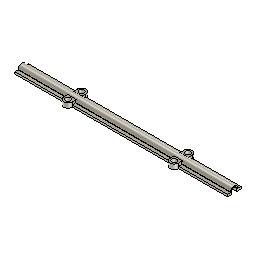
CAN_Cable_Cover v3 (Autodesk Fusion 360 design; units mm, degrees)
Autodesk Fusion 360 part; units mm, degrees
note: some values were not read from the file. Set by a fixed rule: which sketch regions a step uses.
sketch "Sketch1" plane through (0, 0, 0) normal (1, 0, 0) x (0, 1, 0) in component "CAN_Cable_Cover"
  circle A0 centre (0, 2.4) radius 2.4
  line L0 (-2.4, 2.4) -> (-2.4, 0)
  line L1 (0, 2.5) -> (0, 20)
  line L2 (2.4, 2.4) -> (2.4, 0)
  circle A1 centre (0, 2.4) radius 3.4
  line L3 (-3.4, 2.4) -> (-3.4, 0)
  line L4 (-3.4, 0) -> (-2.4, 0)
  line L5 (3.4, 2.4) -> (3.4, 0)
  line L6 (3.4, 0) -> (2.4, 0)
  line L7 (-3.4, 0) -> (-6.4, 0)
  line L8 (-6.4, 0) -> (-6.4, 2)
  line L9 (-6.4, 2) -> (-3.4, 2)
  line L10 (-3.4, 2) -> (-3.4, 0)
  line L11 (6.4, 2) -> (3.4, 2)
  line L12 (6.4, 0) -> (6.4, 2)
  line L13 (3.4, 0) -> (6.4, 0)
  line L14 (3.4, 2) -> (3.4, 0)
  dimension "d1" = 4.8
  dimension "d2" = 1
  dimension "d5" = 3
  dimension "d6" = 2
  constraint vertical origin A0.centre
  constraint coincident origin A0
  constraint coincident A0 L0.start
  constraint tangent A0 L0
  constraint vertical L0
  constraint symmetric L0.start L1 L2.start
  constraint symmetric L0.end L1 L2.end
  constraint coincident A1 L3.start
  constraint tangent A1 L3
  constraint parallel L0 L3
  constraint perpendicular L0 L4
  constraint symmetric L1 L3.start L5.start
  constraint symmetric L1 L3.end L5.end
  constraint horizontal L7
  constraint vertical L8
  constraint horizontal L9
  constraint vertical L10
  constraint symmetric L1 L7.end L12.start
  constraint symmetric L1 L8.end L11.start
  constraint symmetric L1 L9.end L11.end
  measures "d1" diameter of A0
  measures "d5" distance of L3.end L7.end
  measures "d6" distance of L3.end L9.end
extrude "Extrude1" add sketch "Sketch1" along normal mid plane 200 contours A0 L0 L1 A1 L4 | A0 L1 L2 A1 L6 | A1 L3 L4 L10 | A1 L5 L6 L14 | L3 L7 L8 L9 L10 | L5 L11 L12 L13 L14 in component "CAN_Cable_Cover"
sketch "Sketch2" plane through (0, 0, 0) normal (0, 0, -1) x (1, 0, 0) in component "CAN_Cable_Cover"
  line L0 (-100, 2.4) -> (100, 2.4)
  line L1 (100, 2.4) -> (100, 6.4)
  line L2 (100, 6.4) -> (-100, 6.4)
  line L3 (-100, 6.4) -> (-100, 2.4)
  circle A0 centre (-50, 6.4) radius 4
  line L4 (0, -1.75) -> (0, -22.5)
  circle A1 centre (-50, 6.4) radius 2.35
  line L5 (-46, 6.4) -> (-46, 2.4)
  line L6 (-46, 2.4) -> (-50, 2.4)
  line L7 (-54, 6.4) -> (-54, 2.4)
  line L8 (-54, 2.4) -> (-50, 2.4)
  line L9 (1.75, 0) -> (22.5, 0)
  circle A2 centre (-50, -6.4) radius 4
  circle A3 centre (-50, -6.4) radius 2.35
  line L10 (-54, -6.4) -> (-54, -2.4)
  line L11 (-54, -2.4) -> (-50, -2.4)
  line L12 (-46, -2.4) -> (-50, -2.4)
  line L13 (-46, -6.4) -> (-46, -2.4)
  line L14 (46, -2.4) -> (50, -2.4)
  line L15 (54, 6.4) -> (54, 2.4)
  line L16 (54, 2.4) -> (50, 2.4)
  line L17 (46, 6.4) -> (46, 2.4)
  circle A4 centre (50, 6.4) radius 4
  circle A5 centre (50, -6.4) radius 4
  line L18 (54, -6.4) -> (54, -2.4)
  circle A6 centre (50, -6.4) radius 2.35
  line L19 (46, -6.4) -> (46, -2.4)
  circle A7 centre (50, 6.4) radius 2.35
  line L20 (54, -2.4) -> (50, -2.4)
  line L21 (46, 2.4) -> (50, 2.4)
  dimension "d7" = 8
  dimension "d8" = 50
  dimension "d9" = 4.7
  constraint concentric A0 A1
  constraint coincident L2 A0.centre
  constraint coincident A0 L5.start
  constraint tangent A0 L5
  constraint coincident L0 L5.end
  constraint perpendicular L0 L5
  constraint coincident A0 L6.end
  constraint tangent A0 L6
  constraint coincident A0 L7.start
  constraint tangent A0 L7
  constraint coincident L0 L7.end
  constraint perpendicular L0 L7
  constraint symmetric A0 L9 A2
  constraint symmetric A1 L9 A3
  constraint symmetric L5.start L9 L13.start
  constraint symmetric L5.end L9 L12.start
  constraint symmetric L6.end L9 L11.end
  constraint symmetric L7.start L9 L10.start
  constraint symmetric L7.end L9 L10.end
  constraint symmetric A0 L4 A4
  constraint symmetric L4 A1 A7
  constraint symmetric L4 L5.start L17.start
  constraint symmetric L4 L5.end L17.end
  constraint symmetric L4 L6.end L16.end
  constraint symmetric L4 L7.start L15.start
  constraint symmetric L4 L7.end L15.end
  constraint symmetric L4 A2 A5
  constraint symmetric L4 A3 A6
  constraint symmetric L4 L10.start L18.start
  constraint symmetric L4 L10.end L18.end
  constraint symmetric L4 L11.end L14.end
  constraint symmetric L4 L12.start L14.start
  constraint symmetric L4 L13.start L19.start
  measures "d7" diameter of A0
  measures "d8" distance of A0.centre L4
  measures "d9" diameter of A1
extrude "Extrude2" add sketch "Sketch2" against normal blind 4.5 contours L0 A0 L7 L8 | L0 A0 L5 L6 | L2 A0 A1 | L2 A0 A1 | L0 L17 A4 L21 | L2 A4 A7 | L2 A4 A7 | L0 L15 L16 A4 | A2 | A2 L12 L13 | A2 L10 L11 | L14 A5 L19 | A5 L18 L20 | A5 in component "CAN_Cable_Cover"
extrude "Extrude3" cut sketch "Sketch2" against normal blind 16 contours L2 A1 | L2 A7 | A3 | A6 picked at (-50.2862, 5.6708) picked at (49.2594, 5.8292) in component "CAN_Cable_Cover"
component "CAN_Cable_Cover" placed x (1, 0, 0) y (0, 1, 0) z (0, 0, 1) at (0, 0, 0)
equation "d1 = cable_dia"
equation "d2 = tube_thick"
equation "d3 = length"
equation "d4 = 0deg 0'"
equation "d11 = 0deg 0'"
equation "d13 = 0deg 0'"
equation "length = 200 mm"
equation "cable_dia = 4.8 mm"
equation "tube_thick = 1 mm"
named bodies: "CAN_Cable_Cover"
